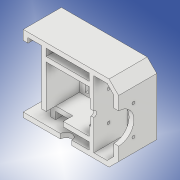
# Autodesk Inventor part: FA001
Saved by Autodesk Inventor 2017 SP1 (Build 210196100, 196)
## iProperties
Created: 2017-06-16
Part Number: FA001
Material: ABS Plastic
Document SubType Name: Modeling
Designer: Zach
Density: 1.06 g/cm^3
Appearance: CR White
Author: Zach
Autodesk Inventor part; units mm, degrees
ref_plane "YZ Plane" through (0, 0, 0) normal (1, 0, 0) x (0, 1, 0)
ref_plane "XZ Plane" through (0, 0, 0) normal (0, 1, 0) x (-1, 0, 0)
ref_plane "XY Plane" through (0, 0, 0) normal (0, 0, 1) x (1, 0, 0)
sketch "Sketch1" plane through (0, 0, 0) normal (0, 0, 1) x (1, 0, 0)
  line L0 (0, 0) -> (100, 0)
  line L1 (100, 0) -> (100, 80) construction
  line L2 (100, 80) -> (0, 80)
  line L3 (0, 80) -> (0, 0)
  line L4 (100, 70) -> (90, 80)
  line L5 (100, 10) -> (90, 0)
  line L6 (100, 70) -> (100, 10)
  line L7 (90, 0) -> (0, 0)
  line L8 (90, 80) -> (0, 80)
  dimension "d0" = 100
  dimension "d1" = 80
  dimension "d15" = 10
  dimension "d16" = 10
  dimension "d17" = 10
  dimension "d18" = 10
  constraints: 18 end point, 4 point on line, 2 collinear, 2 parallel, 1 horizontal, 1 perpendicular
  measures "d0" distance of L2.end L1.end
  measures "d1" distance of L1.end L0.end
  measures "d15" distance of L4.end L1.end
  measures "d16" distance of L4.start L1.end
  measures "d17" distance of L0.end L5.end
  measures "d18" distance of L5.start L0.end
extrude "Extrusion1" add sketch "Sketch1" along normal blind 40
sketch "Sketch2" plane through (0, 0, 40) normal (0, 0, 1) x (1, 0, 0)
  line L0 (90, 80) -> (0, 80) projected
  line L1 (100, 70) -> (90, 80) projected
  line L2 (100, 10) -> (100, 70) projected
  line L3 (90, 0) -> (100, 10) projected
  line L4 (0, 0) -> (90, 0) projected
  line L5 (0, 75) -> (87.9289, 75)
  line L6 (87.9289, 75) -> (95, 67.9289)
  line L7 (95, 67.9289) -> (95, 12.0711)
  line L8 (95, 12.0711) -> (87.9289, 5)
  line L9 (87.9289, 5) -> (0, 5)
  line L10 (0, 80) -> (0, 0) projected
  line L11 (0, 75) -> (0, 5)
  dimension "d19" = 5
  constraints: 12 end point, 1 vertical, 4 other
  measures "d19" distance between parallel lines of L0 L5
extrude "Extrusion2" cut sketch "Sketch2" against normal blind 35 contours L5 L6 L7 L8 L9 L10
sketch "Sketch3" plane through (0, 0, 0) normal (-1, 0, 0) x (0, 0, 1)
  line L0 (0, 80) -> (40, 80)
  line L1 (0, 0) -> (40, 0)
  line L2 (0, 80) -> (10, 80)
  line L3 (10, 80) -> (10, 50)
  line L4 (10, 50) -> (0, 50)
  line L5 (0, 50) -> (0, 80)
  line L6 (40, 80) -> (40, 0)
  line L7 (0, 80) -> (40, 80)
  line L8 (40, 80) -> (40, 70)
  line L9 (40, 70) -> (0, 70)
  line L10 (0, 70) -> (0, 80)
  line L11 (0, 0) -> (40, 0) projected
  line L12 (0, 80) -> (40, 80) projected
  point P0 (20, 0)
  point P1 (20, 80)
  dimension "d7" = 10
  dimension "d8" = 10
  dimension "d11" = 50
  constraints: 22 end point, 4 midpoint, 4 parallel, 2 horizontal, 2 perpendicular, 1 point on line
  measures "d7" distance of L3.end L4.end
  measures "d8" distance of L7.end L8.end
  measures "d11" vertical distance of L1.end L3.end
extrude "Extrusion3" add sketch "Sketch3" against normal blind 5
sketch "Sketch4" plane through (100, 10, 0) normal (1, 0, 0) x (0, 0, -1)
  circle A0 centre (-40, 30) radius 16
  line L0 (-40, 0) -> (-40, 60) projected
  point P0 (66.6667, -50)
  dimension "d12" = 32
  constraints: 1 centre point, 1 coincident, 1 midpoint
  measures "d12" diameter of A0
extrude "Extrusion4" cut sketch "Sketch4" against normal through all
sketch "Sketch5" plane through (0, 0, 5) normal (0, 0, 1) x (1, 0, 0)
  line L0 (74, 75) -> (69, 75)
  line L1 (69, 75) -> (69, 5)
  line L2 (69, 5) -> (74, 5)
  line L3 (74, 5) -> (74, 75)
  line L4 (87.9289, 5) -> (0, 5) projected
  line L5 (5, 75) -> (87.9289, 75) projected
  line L6 (95, 67.9289) -> (95, 56) projected
  point P0 (0, 0)
  dimension "d20" = 5
  dimension "d21" = 21
  constraints: 8 end point, 2 parallel, 2 point on line, 1 horizontal, 1 perpendicular
  measures "d20" distance of L2.end L1.end
  measures "d21" distance between parallel lines of L6 L3
extrude "Extrusion5" add sketch "Sketch5" along normal blind 35
sketch "Sketch6" plane through (69, 5, 5) normal (-1, 0, 0) x (0, 0, 1)
  line L0 (35, 70) -> (35, 0) projected
  circle A0 centre (35, 35) radius 3
  line L1 (19.5, 19.5) -> (50.5, 19.5) construction
  line L2 (50.5, 19.5) -> (50.5, 50.5) construction
  line L3 (50.5, 50.5) -> (19.5, 50.5) construction
  line L4 (19.5, 50.5) -> (19.5, 19.5) construction
  line L5 (19.5, 19.5) -> (50.5, 50.5) construction
  line L6 (50.5, 19.5) -> (19.5, 50.5) construction
  circle A1 centre (19.5, 50.5) radius 1.5
  circle A2 centre (19.5, 19.5) radius 1.5
  point P0 (-5, -5)
  dimension "d24" = 6
  dimension "d25" = 31
  dimension "d26" = 31
  dimension "d27" = 3
  dimension "d28" = 3
  constraints: 12 end point, 3 centre point, 3 midpoint, 2 coincident, 2 parallel, 1 horizontal, 1 perpendicular
  measures "d24" diameter of A0
  measures "d25" distance of L3.end L2.end
  measures "d26" distance of L2.end L1.end
  measures "d27" diameter of A1
  measures "d28" diameter of A2
extrude "Extrusion6" cut sketch "Sketch6" against normal through all
sketch "Sketch7" plane through (69, 5, 5) normal (-1, 0, 0) x (0, 0, 1)
  arc A0 (35, 38) -> (35, 32) centre (35, 35) ccw projected
  circle A1 centre (35, 35) radius 12.5
  point P0 (-5, -5)
  dimension "d31" = 25
  constraints: 1 centre point, 1 coincident
  measures "d31" diameter of A1
extrude "Extrusion7" cut sketch "Sketch7" against normal blind 2
sketch "Sketch8" plane through (0, 0, 5) normal (0, 0, 1) x (1, 0, 0)
  line L0 (69, 17.5) -> (19, 17.5)
  line L1 (19, 17.5) -> (19, 12.5)
  line L2 (19, 12.5) -> (69, 12.5)
  line L3 (69, 12.5) -> (69, 17.5)
  line L4 (69, 27.5) -> (69, 5) projected
  line L5 (69, 67.5) -> (19, 67.5)
  line L6 (19, 67.5) -> (19, 62.5)
  line L7 (19, 62.5) -> (69, 62.5)
  line L8 (69, 62.5) -> (69, 67.5)
  line L9 (19, 62.5) -> (19, 17.5) construction
  line L10 (69, 27.5) -> (69, 52.5) construction
  point P0 (0, 0)
  point P1 (69, 15)
  point P2 (19, 40)
  point P3 (69, 40)
  dimension "d34" = 50
  dimension "d35" = 5
  dimension "d36" = 50
  dimension "d37" = 5
  dimension "d38" = 45
  constraints: 18 end point, 4 parallel, 3 midpoint, 2 horizontal, 2 perpendicular, 1 horizontal alignment, 1 point on line, 1 vertical
  measures "d34" distance of L2.end L1.end
  measures "d35" distance of L1.end L0.end
  measures "d36" distance of L7.end L6.end
  measures "d37" distance of L6.end L5.end
  measures "d38" distance of L0.end L6.end
extrude "Extrusion8" add sketch "Sketch8" along normal blind 35
sketch "Sketch9" plane through (0, 0, 5) normal (0, 0, 1) x (1, 0, 0)
  line L0 (19, 75) -> (24, 75)
  line L1 (24, 75) -> (24, 5)
  line L2 (24, 5) -> (19, 5)
  line L3 (19, 5) -> (19, 75)
  line L4 (5, 75) -> (69, 75) projected
  line L5 (69, 5) -> (0, 5) projected
  point P0 (0, 0)
  point P1 (19, 12.5)
  dimension "d41" = 5
  constraints: 8 end point, 3 point on line, 2 parallel, 1 horizontal, 1 perpendicular
  measures "d41" distance of L1.end L2.end
extrude "Extrusion9" add sketch "Sketch9" along normal blind 35
sketch "Sketch10" plane through (0, 0, 40) normal (0, 0, 1) x (1, 0, 0)
  line L0 (24, 17.5) -> (69, 17.5) projected
  line L1 (19, 5) -> (19, 75) projected
  line L2 (42, 17.5) -> (19, 17.5)
  line L3 (19, 17.5) -> (19, 5)
  line L4 (19, 5) -> (42, 5)
  line L5 (42, 5) -> (42, 17.5)
  point P0 (0, 0)
  dimension "d44" = 23
  constraints: 8 end point, 2 parallel, 1 horizontal, 1 perpendicular, 1 point on line
  measures "d44" distance of L1.start L4.end
extrude "Extrusion10" cut sketch "Sketch10" against normal blind 10
sketch "Sketch11" plane through (0, 0, 5) normal (0, 0, 1) x (1, 0, 0)
  line L0 (30, 59.5) -> (33, 59.5)
  line L1 (33, 59.5) -> (33, 20.5)
  line L2 (33, 20.5) -> (30, 20.5)
  line L3 (30, 20.5) -> (30, 59.5)
  line L4 (24, 62.5) -> (69, 62.5) projected
  line L5 (24, 17.5) -> (42, 17.5) projected
  line L6 (24, 17.5) -> (24, 62.5) projected
  line L7 (36, 59.5) -> (39, 59.5)
  line L8 (39, 59.5) -> (39, 20.5)
  line L9 (39, 20.5) -> (36, 20.5)
  line L10 (36, 20.5) -> (36, 59.5)
  line L11 (42, 59.5) -> (45, 59.5)
  line L12 (45, 59.5) -> (45, 20.5)
  line L13 (45, 20.5) -> (42, 20.5)
  line L14 (42, 20.5) -> (42, 59.5)
  line L15 (48, 59.5) -> (51, 59.5)
  line L16 (51, 59.5) -> (51, 20.5)
  line L17 (51, 20.5) -> (48, 20.5)
  line L18 (48, 20.5) -> (48, 59.5)
  line L19 (54, 59.5) -> (57, 59.5)
  line L20 (57, 59.5) -> (57, 20.5)
  line L21 (57, 20.5) -> (54, 20.5)
  line L22 (54, 20.5) -> (54, 59.5)
  line L23 (60, 59.5) -> (63, 59.5)
  line L24 (63, 59.5) -> (63, 20.5)
  line L25 (63, 20.5) -> (60, 20.5)
  line L26 (60, 20.5) -> (60, 59.5)
  point P0 (0, 0)
  dimension "d47" = 3
  dimension "d48" = 3
  dimension "d49" = 3
  dimension "d50" = 6
  dimension "d53" = 6
  constraints: 48 end point, 2 horizontal, 2 parallel, 1 perpendicular, 40 other
  measures "d47" distance of L1.end L2.end
  measures "d48" distance between parallel lines of L4 L0
  measures "d49" distance between parallel lines of L5 L2
  measures "d50" distance between parallel lines of L6 L3
  measures "d53" distance of L0.start L7.start
extrude "Extrusion11" cut sketch "Sketch11" against normal through all
sketch "Sketch12" plane through (0, 0, 0) normal (0, -1, 0) x (1, 0, 0)
  circle A0 centre (45, 40) radius 6
  line L0 (0, 40) -> (90, 40) projected
  point P0 (0, 0)
  dimension "d60" = 12
  constraints: 1 centre point, 1 coincident, 1 midpoint
  measures "d60" diameter of A0
extrude "Extrusion12" cut sketch "Sketch12" against normal blind 5
body "Solid1"
